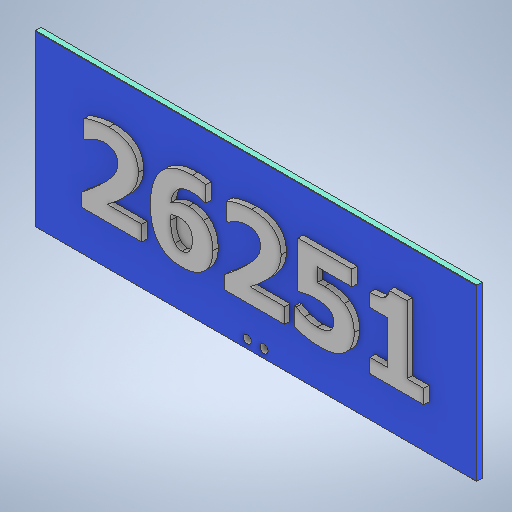
# Autodesk Inventor part: AllianceMkr_BLUE
Saved by Autodesk Inventor 2025.1 (Build 291241000, 241)
## iProperties
Created: 2024-10-13
Part Number: AllianceMkr_BLUE
Material: Generic
Document SubType Name: Modeling
Designer: ishaa
Density: 1 g/cm^3
Appearance: Default
Author: ishaa
Autodesk Inventor part; units mm, degrees
ref_plane "YZ Plane" through (0, 0, 0) normal (1, 0, 0) x (0, 1, 0)
ref_plane "XZ Plane" through (0, 0, 0) normal (0, 1, 0) x (-1, 0, 0)
ref_plane "XY Plane" through (0, 0, 0) normal (0, 0, 1) x (1, 0, 0)
sketch "Sketch4" plane through (0, 0, 0) normal (0, 0, 1) x (1, 0, 0)
  line L0 (82.55, -31.75) -> (-82.55, -31.75)
  line L1 (-82.55, -31.75) -> (-82.55, 31.75)
  line L2 (-82.55, 31.75) -> (82.55, 31.75)
  line L3 (82.55, 31.75) -> (82.55, -31.75)
  line L4 (82.55, -31.75) -> (-82.55, 31.75) construction
  line L5 (-82.55, -31.75) -> (82.55, 31.75) construction
  point P0 (0, 0)
  dimension "d9" = 165.1
  dimension "d10" = 63.5
  constraints: 12 end point, 2 midpoint, 2 parallel, 1 horizontal, 1 perpendicular
  measures "d9" distance of L1.end L2.end
  measures "d10" distance of L0.end L1.end
extrude "Extrusion3" add sketch "Sketch4" along normal blind 2
sketch "Sketch5" plane through (0, 0, 2) normal (0, 0, 1) x (1, 0, 0)
  line L0 (82.55, 31.75) -> (-82.55, 31.75) projected
  line L1 (-82.55, 31.75) -> (-82.55, -31.75) projected
  line L2 (-82.55, -31.75) -> (82.55, -31.75) projected
  line L3 (82.55, -31.75) -> (82.55, 31.75) projected
  line L4 (-82.45, 31.65) -> (82.45, 31.65)
  line L5 (82.45, 31.65) -> (82.45, -31.65)
  line L6 (82.45, -31.65) -> (-82.45, -31.65)
  line L7 (-82.45, -31.65) -> (-82.45, 31.65)
  point P0 (0, 0)
  dimension "d13" = 0.1
  constraints: 8 end point, 3 other
  measures "d13" distance between parallel lines of L0 L4
extrude "Extrusion4" add sketch "Sketch5" along normal blind 0.2 contours L4 L5 L6 L7
sketch "Sketch6" plane through (0, 0, 2.2) normal (0, 0, 1) x (1, 0, 0)
  line L0 (82.45, -31.65) -> (82.45, 31.65) projected
  line L1 (-82.45, 31.65) -> (-82.45, -31.65) projected
  line L2 (82.45, 31.65) -> (-82.45, 31.65) projected
  line L3 (0, 31.65) -> (0, -31.65)
  line L4 (-66.0841, 16.3516) -> (84.0455, 16.3516) construction
  line L5 (84.0455, 16.3516) -> (84.0455, -33.2962) construction
  line L6 (84.0455, -33.2962) -> (-66.0841, -33.2962) construction
  line L7 (-66.0841, -33.2962) -> (-66.0841, 16.3516) construction
  line L8 (-40.5936, -14.7212) -> (-62.9966, -14.7212)
  line L9 (-62.9966, -14.7212) -> (-62.9966, -9.7565)
  spline S0 degree 2 poles (-62.9966, -9.7565) (-60.1561, -7.4841) (-55.6113, -3.4826) (-53.907, -1.6795) knots 0 0 0 1 2 2 2
  spline S1 degree 2 poles (-53.907, -1.6795) (-51.6593, 0.667) (-49.6585, 4.2485) (-49.6585, 6.1257) knots 0 0 0 1 2 2 2
  spline S2 degree 2 poles (-49.6585, 6.1257) (-49.6585, 8.2499) (-52.2027, 10.5224) (-54.4751, 10.5224) knots 0 0 0 1 2 2 2
  spline S3 degree 2 poles (-54.4751, 10.5224) (-55.636, 10.5224) (-57.7108, 9.9542) (-58.7729, 9.5096) knots 0 0 0 1 2 2 2
  spline S4 degree 2 poles (-58.7729, 9.5096) (-59.8103, 9.0403) (-61.2923, 8.0523) (-61.6628, 7.8053) knots 0 0 0 1 2 2 2
  line L10 (-61.6628, 7.8053) -> (-62.2556, 7.8053)
  line L11 (-62.2556, 7.8053) -> (-62.2556, 14.4497)
  spline S5 degree 2 poles (-62.2556, 14.4497) (-60.9712, 15.0672) (-55.4878, 16.3516) (-52.9437, 16.3516) knots 0 0 0 1 2 2 2
  spline S6 degree 2 poles (-52.9437, 16.3516) (-47.5096, 16.3516) (-41.9274, 11.5104) (-41.9274, 7.1384) knots 0 0 0 1 2 2 2
  spline S7 degree 2 poles (-41.9274, 7.1384) (-41.9274, 4.4461) (-44.4715, -0.7409) (-47.4108, -3.7049) knots 0 0 0 1 2 2 2
  spline S8 degree 2 poles (-47.4108, -3.7049) (-49.2633, -5.5328) (-52.7461, -8.3733) (-53.5118, -8.9661) knots 0 0 0 1 2 2 2
  line L12 (-53.5118, -8.9661) -> (-40.5936, -8.9661)
  line L13 (-40.5936, -8.9661) -> (-40.5936, -14.7212)
  spline S9 degree 2 poles (-14.0656, -4.3471) (-14.0656, -9.1637) (-20.1665, -15.3634) (-25.5018, -15.3634) knots 0 0 0 1 2 2 2
  spline S10 degree 2 poles (-25.5018, -15.3634) (-28.1694, -15.3634) (-32.3437, -13.832) (-33.801, -12.3253) knots 0 0 0 1 2 2 2
  spline S11 degree 2 poles (-33.801, -12.3253) (-35.53, -10.5716) (-37.3826, -5.0141) (-37.3826, -1.1361) knots 0 0 0 1 2 2 2
  spline S12 degree 2 poles (-37.3826, -1.1361) (-37.3826, 2.8653) (-35.6535, 9.0897) (-33.7022, 11.4857) knots 0 0 0 1 2 2 2
  spline S13 degree 2 poles (-33.7022, 11.4857) (-31.8497, 13.7581) (-25.8229, 16.3269) (-21.698, 16.3269) knots 0 0 0 1 2 2 2
  spline S14 degree 2 poles (-21.698, 16.3269) (-20.1912, 16.3269) (-17.1778, 15.9317) (-16.6344, 15.8082) knots 0 0 0 1 2 2 2
  line L14 (-16.6344, 15.8082) -> (-16.6344, 9.8307)
  line L15 (-16.6344, 9.8307) -> (-17.1778, 9.8307)
  spline S15 degree 2 poles (-17.1778, 9.8307) (-17.7212, 10.1024) (-20.1912, 10.7694) (-21.7721, 10.7694) knots 0 0 0 1 2 2 2
  spline S16 degree 2 poles (-21.7721, 10.7694) (-25.3536, 10.7694) (-29.2562, 6.9902) (-29.7255, 3.4828) knots 0 0 0 1 2 2 2
  spline S17 degree 2 poles (-29.7255, 3.4828) (-28.2188, 4.4461) (-25.1313, 5.5823) (-23.18, 5.5823) knots 0 0 0 1 2 2 2
  spline S18 degree 2 poles (-23.18, 5.5823) (-21.5251, 5.5823) (-18.6351, 4.6931) (-17.5236, 3.8533) knots 0 0 0 1 2 2 2
  spline S19 degree 2 poles (-17.5236, 3.8533) (-15.9428, 2.643) (-14.0656, -1.2843) (-14.0656, -4.3471) knots 0 0 0 1 2 2 2
  spline S20 degree 2 poles (-22.9824, -8.9414) (-22.3896, -8.2004) (-21.7474, -6.4714) (-21.7474, -4.7176) knots 0 0 0 1 2 2 2
  spline S21 degree 2 poles (-21.7474, -4.7176) (-21.7474, -3.2356) (-22.4884, -1.309) (-23.1553, -0.7409) knots 0 0 0 1 2 2 2
  spline S22 degree 2 poles (-23.1553, -0.7409) (-23.8469, -0.1481) (-25.5512, 0.2718) (-26.5145, 0.2718) knots 0 0 0 1 2 2 2
  spline S23 degree 2 poles (-26.5145, 0.2718) (-27.3296, 0.2718) (-29.0092, -0.1481) (-29.7502, -0.4445) knots 0 0 0 1 2 2 2
  spline S24 degree 2 poles (-29.7502, -0.4445) (-29.7502, -0.6421) (-29.7996, -1.5807) (-29.7996, -2.297) knots 0 0 0 1 2 2 2
  spline S25 degree 2 poles (-29.7996, -2.297) (-29.7996, -4.94) (-28.8857, -8.1263) (-28.1694, -8.9414) knots 0 0 0 1 2 2 2
  spline S26 degree 2 poles (-28.1694, -8.9414) (-27.6507, -9.6083) (-26.2675, -10.1764) (-25.5265, -10.1764) knots 0 0 0 1 2 2 2
  spline S27 degree 2 poles (-25.5265, -10.1764) (-24.909, -10.1764) (-23.4764, -9.5589) (-22.9824, -8.9414) knots 0 0 0 1 2 2 2
  line L16 (12.8082, -14.7212) -> (-9.5949, -14.7212)
  line L17 (-9.5949, -14.7212) -> (-9.5949, -9.7565)
  spline S28 degree 2 poles (-9.5949, -9.7565) (-6.7544, -7.4841) (-2.2095, -3.4826) (-0.5052, -1.6795) knots 0 0 0 1 2 2 2
  spline S29 degree 2 poles (-0.5052, -1.6795) (1.7425, 0.667) (3.7432, 4.2485) (3.7432, 6.1257) knots 0 0 0 1 2 2 2
  spline S30 degree 2 poles (3.7432, 6.1257) (3.7432, 8.2499) (1.1991, 10.5224) (-1.0733, 10.5224) knots 0 0 0 1 2 2 2
  spline S31 degree 2 poles (-1.0733, 10.5224) (-2.2342, 10.5224) (-4.309, 9.9542) (-5.3711, 9.5096) knots 0 0 0 1 2 2 2
  spline S32 degree 2 poles (-5.3711, 9.5096) (-6.4086, 9.0403) (-7.8906, 8.0523) (-8.2611, 7.8053) knots 0 0 0 1 2 2 2
  line L18 (-8.2611, 7.8053) -> (-8.8539, 7.8053)
  line L19 (-8.8539, 7.8053) -> (-8.8539, 14.4497)
  spline S33 degree 2 poles (-8.8539, 14.4497) (-7.5695, 15.0672) (-2.086, 16.3516) (0.4581, 16.3516) knots 0 0 0 1 2 2 2
  spline S34 degree 2 poles (0.4581, 16.3516) (5.8921, 16.3516) (11.4744, 11.5104) (11.4744, 7.1384) knots 0 0 0 1 2 2 2
  spline S35 degree 2 poles (11.4744, 7.1384) (11.4744, 4.4461) (8.9302, -0.7409) (5.9909, -3.7049) knots 0 0 0 1 2 2 2
  spline S36 degree 2 poles (5.9909, -3.7049) (4.1384, -5.5328) (0.6557, -8.3733) (-0.11, -8.9661) knots 0 0 0 1 2 2 2
  line L20 (-0.11, -8.9661) -> (12.8082, -8.9661)
  line L21 (12.8082, -8.9661) -> (12.8082, -14.7212)
  spline S37 degree 2 poles (38.8174, -4.3965) (38.8174, -6.7925) (37.1872, -10.8433) (35.5817, -12.3006) knots 0 0 0 1 2 2 2
  spline S38 degree 2 poles (35.5817, -12.3006) (33.9762, -13.7579) (29.5796, -15.3634) (26.3686, -15.3634) knots 0 0 0 1 2 2 2
  spline S39 degree 2 poles (26.3686, -15.3634) (22.9599, -15.3387) (18.0693, -14.2272) (16.4638, -13.5109) knots 0 0 0 1 2 2 2
  line L22 (16.4638, -13.5109) -> (16.4638, -6.8666)
  line L23 (16.4638, -6.8666) -> (17.1554, -6.8666)
  spline S40 degree 2 poles (17.1554, -6.8666) (17.7482, -7.1877) (19.1808, -8.0275) (20.3417, -8.4721) knots 0 0 0 1 2 2 2
  spline S41 degree 2 poles (20.3417, -8.4721) (21.4285, -8.892) (23.6762, -9.4601) (25.0348, -9.4601) knots 0 0 0 1 2 2 2
  spline S42 degree 2 poles (25.0348, -9.4601) (26.2204, -9.4601) (28.9868, -8.8673) (29.8266, -8.0769) knots 0 0 0 1 2 2 2
  spline S43 degree 2 poles (29.8266, -8.0769) (30.4441, -7.4594) (31.1357, -5.9527) (31.1357, -4.6929) knots 0 0 0 1 2 2 2
  spline S44 degree 2 poles (31.1357, -4.6929) (31.1357, -3.6061) (30.2465, -2.0747) (29.5302, -1.6054) knots 0 0 0 1 2 2 2
  spline S45 degree 2 poles (29.5302, -1.6054) (28.4928, -0.9138) (25.5288, -0.5186) (24.4666, -0.5186) knots 0 0 0 1 2 2 2
  spline S46 degree 2 poles (24.4666, -0.5186) (22.787, -0.5186) (19.6007, -1.062) (18.4398, -1.3584) knots 0 0 0 1 2 2 2
  line L24 (18.4398, -1.3584) -> (17.7729, -1.3584)
  line L25 (17.7729, -1.3584) -> (17.7729, 15.7588)
  line L26 (17.7729, 15.7588) -> (37.9776, 15.7588)
  line L27 (37.9776, 15.7588) -> (37.9776, 10.0036)
  line L28 (37.9776, 10.0036) -> (25.0101, 10.0036)
  line L29 (25.0101, 10.0036) -> (25.0101, 4.9401)
  spline S47 degree 2 poles (25.0101, 4.9401) (25.6276, 4.9895) (27.3319, 5.0389) (27.8012, 5.0389) knots 0 0 0 1 2 2 2
  spline S48 degree 2 poles (27.8012, 5.0389) (29.9995, 5.0389) (33.7045, 4.1497) (35.1618, 3.2358) knots 0 0 0 1 2 2 2
  spline S49 degree 2 poles (35.1618, 3.2358) (36.8908, 2.0996) (38.8174, -1.6795) (38.8174, -4.3965) knots 0 0 0 1 2 2 2
  line L30 (64.8514, -14.7212) -> (44.7208, -14.7212)
  line L31 (44.7208, -14.7212) -> (44.7208, -9.4107)
  line L32 (44.7208, -9.4107) -> (51.1428, -9.4107)
  line L33 (51.1428, -9.4107) -> (51.1428, 6.7185)
  line L34 (51.1428, 6.7185) -> (44.7208, 6.7185)
  line L35 (44.7208, 6.7185) -> (44.7208, 11.6833)
  spline S50 degree 2 poles (44.7208, 11.6833) (46.1287, 11.6833) (48.9198, 12.0538) (49.7596, 12.449) knots 0 0 0 1 2 2 2
  spline S51 degree 2 poles (49.7596, 12.449) (50.7229, 12.943) (51.8097, 14.5979) (51.9085, 15.8329) knots 0 0 0 1 2 2 2
  line L36 (51.9085, 15.8329) -> (58.5776, 15.8329)
  line L37 (58.5776, 15.8329) -> (58.5776, -9.4107)
  line L38 (58.5776, -9.4107) -> (64.8514, -9.4107)
  line L39 (64.8514, -9.4107) -> (64.8514, -14.7212)
  point P0 (0, 0)
  constraints: 2 end point, 1 horizontal, 1 midpoint, 1 vertical, 2 other
emboss "Emboss1" sketch "Sketch6" operation add depth 2 direction (0, 0, -1) contours S33 S34 S35 S36 L3 S29 S30 | L3 S30 S31 S32 L18 L19 S33 | L3 S36 L20 L16 L17 S28 S29 | L20 L21 L16 L3 | L8 L9 S0 S1 S2 S3 S4 L10 L11 S5 S6 S7 S8 L12 L13 | S9 S10 S11 S12 S13 S14 L14 L15 S15 S16 S17 S18 S19 | S37 S38 S39 L22 L23 S40 S41 S42 S43 S44 S45 S46 L24 L25 L26 L27 L28 L29 S47 S48 S49 | L30 L31 L32 L33 L34 L35 S50 S51 L36 L37 L38 L39
sketch "Sketch7" plane through (0, 0, 2.2) normal (0, 0, 1) x (1, 0, 0)
  circle A0 centre (-3.1464, -28.4734) radius 1.5
  line L0 (0, -19.2895) -> (0, -31.65) construction
  line L1 (-82.45, -31.65) -> (82.45, -31.65) construction
  circle A1 centre (3.1464, -28.4734) radius 1.5
  point P0 (0, 0)
  dimension "d21" = 3
  dimension "d22" = 3.1464
  dimension "d23" = 9.7079
  dimension "d24" = 4.4711
  constraints: 2 centre point, 2 end point, 1 midpoint, 1 symmetric about line, 1 vertical, 1 other
  measures "d21" diameter of A0
  measures "d22" distance from line of A1.centre L0
  measures "d23" distance of L0.start A1.centre
  measures "d24" distance of L0.end A1.centre
extrude "Extrusion5" cut sketch "Sketch7" against normal blind 12700
body "Solid2"
